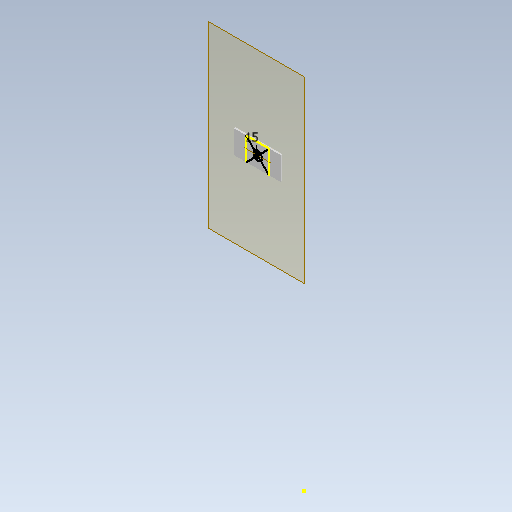
# Autodesk Inventor part: victum
Saved by Autodesk Inventor 2020 (Build 240168000, 168)
## iProperties
Created: 2022-10-11
Part Number: victum
Material: Типовые
Document SubType Name: Modeling
Designer: akapu
Density: 1 g/cm^3
Appearance: По умолчанию
Author: akapu
Autodesk Inventor part; units mm, degrees
ref_plane "YZ Plane" through (0, 0, 0) normal (1, 0, 0) x (0, 1, 0)
ref_plane "XZ Plane" through (0, 0, 0) normal (0, 1, 0) x (-1, 0, 0)
ref_plane "XY Plane" through (0, 0, 0) normal (0, 0, 1) x (1, 0, 0)
ref_plane "РабПлоскость1" through (0, 10, -310) normal (0, 0, 1) x (1, 0, 0)
sketch "Эскиз1" plane through (0, 10, -310) normal (0, 0, 1) x (1, 0, 0)
  line L0 (-10, 590) -> (-160, 590) projected
  line L1 (-160, 310) -> (-160, 590) projected
  line L2 (-160, 310) -> (-10, 310) projected
  line L3 (-10, 590) -> (-10, 310) projected
  line L4 (-10, 450) -> (-80, 450)
  line L5 (-100, 430) -> (-60, 430)
  line L6 (-60, 430) -> (-60, 470)
  line L7 (-60, 470) -> (-100, 470)
  line L8 (-100, 470) -> (-100, 430)
  line L9 (-100, 430) -> (-60, 470) construction
  line L10 (-60, 430) -> (-100, 470) construction
  point P0 (0, -10)
  dimension "d0" = 70
  dimension "d1" = 40
  dimension "d2" = 40
  constraints: 14 end point, 3 midpoint, 2 parallel, 2 perpendicular, 1 horizontal
  measures "d0" distance of L4.start L4.end
  measures "d1" distance of L7.end L6.end
  measures "d2" distance of L6.end L5.end
extrude "Выдавливание1" add sketch "Эскиз1" along normal blind 3 contours L6 L5 L8 L7
ref_plane "РабПлоскость2" through (-100, 460, -310) normal (0, 1, 0) x (1, 0, 0)
sketch "Эскиз2" plane through (0, 10, -307) normal (0, 0, 1) x (1, 0, 0)
  line L0 (-60, 470) -> (-100, 470) projected
  line L1 (-100, 470) -> (-100, 430) projected
  line L2 (-60, 470) -> (-100, 430)
  line L3 (-60, 430) -> (-60, 470) projected
  line L4 (-60, 430) -> (-100, 470)
  circle A0 centre (-80, 450) radius 7.5
  point P0 (0, -10)
  dimension "d5" = 15
  constraints: 4 end point, 1 centre point, 1 midpoint
  measures "d5" diameter of A0
sketch "Эскиз3" plane through (0, 10, -310) normal (0, 0, -1) x (-1, 0, 0)
  line L0 (100, 430) -> (60, 430) projected
  line L1 (60, 430) -> (40, 430)
  line L2 (40, 430) -> (120, 430)
  line L3 (120, 430) -> (120, 470)
  line L4 (120, 470) -> (40, 470)
  line L5 (40, 470) -> (40, 430)
  point P0 (0, -10)
  dimension "d6" = 20
  dimension "d7" = 80
  constraints: 10 end point, 2 horizontal, 2 parallel, 1 perpendicular
  measures "d6" distance of L0.end L1.end
  measures "d7" distance of L4.end L3.end
extrude "Выдавливание2" add sketch "Эскиз3" against normal blind 3
